Motor Coupling 5mm v3 (Autodesk Fusion 360 design; units mm, degrees)
Autodesk Fusion 360 part; units mm, degrees
sketch "Sketch1" plane through (0, 0, 0) normal (0, 0, 1) x (1, 0, 0)
  circle A0 centre (0, 0) radius 11
  circle A1 centre (0, 0) radius 2.5
  circle A2 centre (0, 0) radius 8 construction
  circle A3 centre (0, 8) radius 1.5
  line L0 (0, 0) -> (0, 11) construction
  circle A4 centre (-8, 0) radius 1.5
  circle A5 centre (0, -8) radius 1.5
  circle A6 centre (8, 0) radius 1.5
  dimension "d1" = 22
  dimension "d2" = 5
  dimension "d3" = 16
  dimension "d4" = 3
  dimension "d6" = 360
  constraint coincident A0.centre A1.centre
  constraint concentric A0 A1
  constraint concentric A1 A2
  constraint coincident A2 A3.centre
  constraint coincident A0 L0.end
  constraint vertical L0
  measures "d1" diameter of A0
  measures "d2" diameter of A1
  measures "d3" diameter of A2
  measures "d4" diameter of A3
extrude "Extrude1" add sketch "Sketch1" along normal blind 2
sketch "Sketch2" plane through (0, 0, 2) normal (0, 0, 1) x (-1, 0, 0)
  circle A0 centre (0, 0) radius 2.5
  circle A1 centre (8, 0) radius 1.5
  circle A2 centre (0, -8) radius 1.5
  circle A3 centre (0, 8) radius 1.5
  circle A4 centre (0, 0) radius 11
  circle A5 centre (0, 0) radius 5
  circle A6 centre (-8, 0) radius 1.5
  dimension "d9" = 10
  constraint concentric A0 A5
  measures "d9" diameter of A5
extrude "Extrude2" add sketch "Sketch2" along normal blind 10 contours A5
